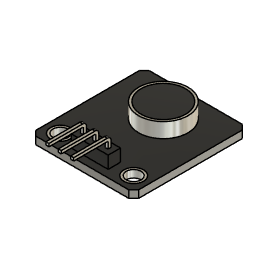
Vibration-Motor v1 (Autodesk Fusion 360 design; units mm, degrees)
Autodesk Fusion 360 part; units mm, degrees
sketch "Sketch1" plane through (0, 0, 0) normal (0, 0, 1) x (1, 0, 0)
  line L0 (9.4329, 11.4921) -> (-9.4329, 11.4921)
  line L1 (-10.425, 10.5) -> (-10.425, -10.5)
  line L2 (-9.425, -11.5) -> (9.425, -11.5)
  line L3 (10.425, -10.5) -> (10.425, 10.5)
  line L4 (9.9495, 10.9755) -> (-9.9495, -10.9755) construction
  line L5 (-9.9495, 10.9755) -> (9.9495, -10.9755) construction
  circle A0 centre (-7.425, -8.5) radius 2
  circle A1 centre (7.425, -8.5) radius 2
  circle A2 centre (-7.425, -8.5) radius 1.5
  circle A3 centre (7.425, -8.5) radius 1.5
  line L6 (0, 11.4921) -> (0, -11.5)
  line L7 (-9.425, -11.5) -> (-10.425, -10.5)
  line L8 (9.425, -11.5) -> (10.425, -10.5)
  line L9 (-10.425, 10.5) -> (-9.4329, 11.4921)
  line L10 (9.4329, 11.4921) -> (10.425, 10.5)
  circle A4 centre (0.425, 4.505) radius 5
  circle A5 centre (0.425, 4.505) radius 4.5
  line L11 (3.75, -10) -> (-3.75, -10)
  line L12 (-3.75, -10) -> (-3.75, -7.5)
  line L13 (-3.75, -7.5) -> (3.75, -7.5)
  line L14 (3.75, -7.5) -> (3.75, -10)
  line L15 (3.75, -10) -> (-3.75, -7.5) construction
  line L16 (-3.75, -10) -> (3.75, -7.5) construction
  point P0 (0, -8.75)
  dimension "d3" = 4
  dimension "d6" = -0.5
  dimension "d8" = 3
  dimension "d9" = 3
  dimension "d18" = 10
  dimension "d19" = -0.5
  dimension "d20" = 7
  dimension "d21" = 10
  dimension "d22" = 7.5
  dimension "d23" = 2.5
  dimension "d24" = 1.5
  constraint horizontal L0
  constraint perpendicular L0 L1
  constraint parallel L0 L2
  constraint parallel L1 L3
  constraint coincident L4 origin
  constraint coincident L5 origin
  constraint equal A0 A1
  constraint concentric A1 A3
  constraint equal A2 A3
  constraint symmetric A2 A3 L6
  constraint coincident L8 L5.end
  constraint coincident L2 L6.end
  constraint coincident L7 L4.end
  constraint coincident L10 L4.start
  constraint coincident L0 L6.start
  constraint coincident L9 L5.start
  constraint horizontal L11
  constraint perpendicular L11 L12
  constraint parallel L11 L13
  constraint parallel L12 L14
  constraint coincident L15 P0
  constraint coincident L16 P0
  constraint coincident L6 P0
  measures "d3" diameter of A0
  measures "d8" distance of L1 A0.centre
  measures "d9" distance of L2 A0.centre
  measures "d18" diameter of A4
  measures "d20" distance of L6.start A4.centre
  measures "d21" distance of L3 A4.centre
  measures "d22" distance of L12.end L13.end
  measures "d23" distance of L11.end L12.end
  measures "d24" distance of L2 L11
extrude "Extrude1" add sketch "Sketch1" along normal blind 1.5 contours L0 L2 L3 L6 L8 L10 A4 L11 L13 L14 | L0 L1 L2 L6 L7 L9 A4 L11 L12 L13 | L6 A4 A5 | L6 A4 A5 | L6 A5 | L6 A5 | L6 L11 L13 L14 | L6 L11 L12 L13 | A0 | A1 makes body 1
split "Split1" by curves path "Sketch1" along A0 A1 bodies 1 makes body 2 at (8.9231, -8.5748, 1) makes body 3 at (0, -0.7935, 0)
extrude "Extrude2" add sketch "Sketch1" along normal blind 3 from surface at 1.5 separate body contours L6 A4 A5 | L6 A4 A5 | L6 A5 | L6 A5 makes body 4
split "Split2" by curves path "Sketch1" along A5 bodies 4 makes body 5 at (-4.4225, 5.7305, 3.5)
extrude "Extrude3" add sketch "Sketch1" along normal blind 2.5 from surface at 1.5 separate body contours L6 L11 L13 L14 | L6 L11 L12 L13 makes body 6
sketch "Sketch2" plane through (0, 0, 4) normal (0, 0, 1) x (-1, 0, 0)
  line L0 (-3.75, 10) -> (-3.75, 7.5)
  line L1 (-3.75, 7.5) -> (3.75, 7.5)
  line L2 (3.75, 7.5) -> (3.75, 10)
  line L3 (3.75, 10) -> (-3.75, 10)
  line L4 (2.9, 8.35) -> (2.3, 8.35)
  line L5 (2.3, 8.35) -> (2.3, 8.95)
  line L6 (2.3, 8.95) -> (2.9, 8.95)
  line L7 (2.9, 8.95) -> (2.9, 8.35)
  line L8 (3.75, 10) -> (3.75, 7.5)
  line L9 (3.75, 7.5) -> (-3.75, 7.5)
  dimension "d33" = 0.6
  dimension "d34" = 0.6
  dimension "d35" = 0.85
  dimension "d36" = 0.85
  constraint horizontal L4
  constraint vertical L5
  constraint horizontal L6
  constraint vertical L7
  measures "d33" distance of L4.start L4.end
  measures "d34" distance of L4.start L6.end
  measures "d35" distance of L7 L8
  measures "d36" distance of L4 L9
extrude "Extrude4" add sketch "Sketch2" along normal blind 2 separate body contours L4 L5 L6 L7 makes body 7
sketch "Sketch3" plane through (0, -8.95, 0) normal (0, -1, 0) x (1, 0, 0)
  line L0 (-2.3, 4) -> (-2.3, 6)
  line L1 (-2.3, 6) -> (-2.9, 6)
  line L2 (-2.9, 6) -> (-2.9, 4)
  line L3 (-2.9, 5.4) -> (-2.3, 5.4)
  line L4 (-2.9, 4) -> (-2.3, 4)
  dimension "d39" = 0.6
  constraint coincident L2 L3.start
  constraint coincident L0 L3.end
  constraint perpendicular L0 L3
  measures "d39" distance of L1 L3
extrude "Extrude5" add sketch "Sketch3" along normal blind 7 contours L0 L1 L2 L3 bodies 6 7
fillet "Fillet1" radius 0.75 1 edges at (-2.6, -8.35, 6) on bodies 7
fillet "Fillet1" radius 0.15 1 edges at (-2.6, -8.95, 5.4) on bodies 7
pattern_linear "R-Pattern1" count 3 spacing 2.5 along (1, 0, 0) of bodies 7 makes body 8 at (0.2, -13.6667, 5.6) makes body 9 at (2.7, -13.6667, 5.6)
